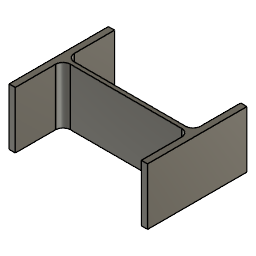
H-244×175×7×11 (Autodesk Fusion 360 design; units mm, degrees)
Autodesk Fusion 360 part; units mm, degrees
sketch "スケッチ1" plane through (0, 0, 0) normal (0, 0, 1) x (1, 0, 0)
  line L0 (24, -3.5) -> (220, -3.5)
  line L1 (220, 3.5) -> (24, 3.5)
  line L2 (11, 16.5) -> (11, 87.5)
  line L3 (0, 87.5) -> (0, -87.5)
  line L4 (11, -87.5) -> (11, -16.5)
  line L5 (0, -87.5) -> (11, -87.5)
  line L6 (11, 87.5) -> (0, 87.5)
  line L7 (244, -87.5) -> (244, 87.5)
  line L8 (233, 87.5) -> (233, 16.5)
  line L9 (233, -16.5) -> (233, -87.5)
  line L10 (233, -87.5) -> (244, -87.5)
  line L11 (244, 87.5) -> (233, 87.5)
  arc A0 (24, -3.5) -> (11, -16.5) centre (24, -16.5) ccw
  arc A1 (11, 16.5) -> (24, 3.5) centre (24, 16.5) ccw
  arc A2 (220, 3.5) -> (233, 16.5) centre (220, 16.5) ccw
  arc A3 (233, -16.5) -> (220, -3.5) centre (220, -16.5) ccw
extrude "押し出し1" add sketch "スケッチ1" along normal blind 100
